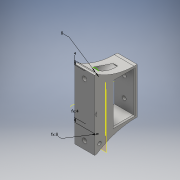
# Autodesk Inventor part: espaceur_20mm_v3
Saved by Autodesk Inventor 2016 (Build 200138000, 138)
## iProperties
Created: 2018-02-21
Part Number: espaceur_20mm_v3
Material: Generic
Document SubType Name: Modeling
Designer: mbouhier
Density: 1 g/cm^3
Appearance: Default
Author: mbouhier
Autodesk Inventor part; units mm, degrees
note: some values were not read from the file. Chosen so that the rebuilt part matches the saved one: sketch regions of "Extrusion1"; direction of "Hole1".
ref_plane "YZ Plane" through (0, 0, 0) normal (1, 0, 0) x (0, 1, 0)
ref_plane "XZ Plane" through (0, 0, 0) normal (0, 1, 0) x (-1, 0, 0)
ref_plane "XY Plane" through (0, 0, 0) normal (0, 0, 1) x (1, 0, 0)
sketch "Sketch1" plane through (0, 0, 0) normal (1, 0, 0) x (0, 1, 0)
  line L0 (0, 0) -> (0, -35.075)
  line L1 (0, -35.075) -> (2, -35.075)
  line L2 (19.925, 20.075) -> (40.075, 20.075)
  line L3 (40.075, 20.075) -> (40.075, -20.075)
  line L4 (40.075, -20.075) -> (19.925, -20.075)
  line L5 (19.925, -20.075) -> (19.925, 20.075)
  line L6 (19.925, 20.075) -> (40.075, -20.075) construction
  line L7 (40.075, 20.075) -> (19.925, -20.075) construction
  line L8 (16.925, 23.075) -> (43.075, 23.075)
  line L9 (43.075, 23.075) -> (43.075, -23.075)
  line L10 (43.075, -23.075) -> (16.925, -23.075)
  line L11 (16.925, -23.075) -> (16.925, 23.075)
  line L12 (16.925, 23.075) -> (43.075, -23.075) construction
  line L13 (43.075, 23.075) -> (16.925, -23.075) construction
  line L14 (0, 0) -> (0, 35.075)
  line L15 (0, 35.075) -> (2, 35.075)
  arc A0 (2, 35.075) -> (43.075, 23.075) centre (41.5508, 94.1558) ccw
  arc A1 (43.075, -23.075) -> (2, -35.075) centre (42.3004, -96.7217) ccw
  line L16 (-8.615, 0) -> (51.69, 0) projected
  point P0 (20, 0)
  point P1 (40.1, 0)
  point P2 (30, 0)
  point P3 (30, 23.075)
  point P4 (30.025, -23.075)
  point P5 (30, 0)
  dimension "d0" = 35.075
  dimension "d1" = 2
  dimension "d2" = 20
  dimension "d4" = 20.15
  dimension "d5" = 40.15
  dimension "d6" = 46.15
  dimension "d7" = 26.15
  dimension "d8" = 35.075
  constraints: 32 end point, 6 midpoint, 4 parallel, 4 point on circle, 3 horizontal, 3 perpendicular, 2 centre point, 2 point on line, 2 vertical
  measures "d0" distance of L0.start L0.end
  measures "d1" distance of L0.end L1.end
  measures "d2" distance of point (20, 0) L0.start
  measures "d4" distance of L3.end L4.end
  measures "d5" distance of L2.end L3.end
  measures "d6" distance of L8.end L9.end
  measures "d7" distance of L8.start L8.end
  measures "d8" distance of L0.start L14.end
extrude "Extrusion1" add sketch "Sketch1" along normal blind 20 contours L10 L11 L16 L5 L4 L3 L9 | L16 L11 L10 A1 L1 L0 | L14 L15 A0 L8 L11 L16 | L11 L8 A0 L9 L16 L3 L2 L5 | L8 A0
sketch "Sketch2" plane through (0, 43.075, 23.075) normal (0, 1, 0) x (1, 0, 0)
  line L0 (0, 46.15) -> (0, 0) projected
  line L1 (0, 0) -> (20, 0) projected
  line L2 (20, 46.15) -> (20, 0) projected
  line L3 (0, 46.15) -> (20, 46.15) projected
  line L4 (0, 3) -> (20, 3) projected
  line L5 (0, 3) -> (20, 3) projected
  point P0 (0, 23.075)
  point P1 (10, 13.05)
  point P2 (10, 33.05)
  dimension "d33" = 20
  dimension "d34" = 10.05
  measures "d33" distance of point (10, 33.05) point (10, 13.05)
  measures "d34" distance from line of point (10, 13.05) L4
hole "Hole1" at (10, 43.075, 10.025) at (10, 43.075, -9.975) direction (0, -1, 0) diameter 4 end up to surface
ref_plane "Work Plane1" through (0, 11, -35.075) normal (0, -1, 0) x (1, 0, 0)
sketch "Sketch3" plane through (0, 11, -35.075) normal (0, -1, 0) x (1, 0, 0)
  circle A0 centre (10, 45.1) radius 2 projected
  line L0 (0, 12) -> (0, 58.15) projected
  line L1 (0, 58.15) -> (20, 58.15) projected
  line L2 (20, 12) -> (20, 58.15) projected
  line L3 (0, 12) -> (20, 12) projected
  line L4 (0, 55.15) -> (0, 15) projected
  line L5 (0, 55.15) -> (20, 55.15) projected
  line L6 (20, 15) -> (20, 55.15) projected
  line L7 (0, 15) -> (20, 15) projected
  circle A1 centre (10, 62.15) radius 4
  circle A2 centre (10, 8) radius 4
  point P0 (0, 35.075)
  dimension "d19" = 4
  dimension "d20" = 4
  dimension "d30" = 8
  dimension "d31" = 8
  constraints: 2 centre point, 2 coincident
  measures "d19" distance from line of point (10, 62.15) L1
  measures "d20" distance from line of L3 point (10, 8)
  measures "d30" diameter of A1
  measures "d31" diameter of A2
extrude "Extrusion2" cut sketch "Sketch3" against normal blind 20 contours A1 | A2
hole "Hole2" at (10, 11, 27.075) at (10, 11, -27.075) direction (0, -1, 0) diameter 4.5 end through all
chamfer "Chamfer1" distance 1 angle 45 4 edges at (20, 40.075, 0) (20, 30, 20.075) (20, 19.925, 0) (20, 30, -20.075)
sketch "Sketch4" plane through (20, 0, 0) normal (1, 0, 0) x (0, 0, -1)
  line L0 (0, -8.615) -> (0, 51.69) projected
  line L1 (-35.075, 0) -> (35.075, 0) projected
  line L2 (0, 0) -> (2, 2)
  line L3 (2, 2) -> (-2, 2)
  line L4 (-2, 2) -> (0, 0)
  constraints: 6 end point, 1 horizontal, 1 perpendicular
extrude "Extrusion3" add sketch "Sketch4" along normal blind 0.4
sketch "Sketch5" plane through (20, 0, 0) normal (1, 0, 0) x (0, 0, -1)
  line L0 (0, 0) -> (35.075, 0) projected
  line L1 (35.075, 0) -> (35.075, 2) projected
  point P0 (27.075, 5)
  dimension "d42" = 5
  dimension "d43" = 8
  measures "d42" distance from line of point (27.075, 5) L0
  measures "d43" distance from line of point (27.075, 5) L1
hole "Hole3" at (20, 5, -27.075) direction (-1, 0, 0) diameter 3.5 depth 5
equation "\"d8\" = d0"
equation "\"d20\" = d19"
equation "\"d31\" = d30"
body "Solid1"
